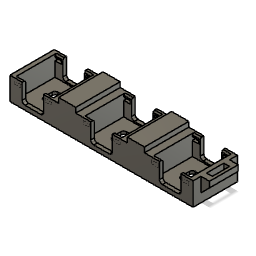
Magnet_Storage_Drawer (Autodesk Fusion 360 design; units mm, degrees)
Autodesk Fusion 360 part; units mm, degrees
sketch "base" plane through (0, 0, 0) normal (0, 1, 0) x (1, 0, 0)
  line L0 (-64, 15.5) -> (64, 15.5)
  line L1 (64, 15.5) -> (64, -15.5)
  line L2 (64, -15.5) -> (-64, -15.5)
  line L3 (-64, -15.5) -> (-64, 15.5)
  line L4 (64, 0) -> (-64, 0) construction
  line L5 (0, 15.5) -> (0, -15.5) construction
  line L6 (-61, 13) -> (-35, 13)
  line L7 (-35, 13) -> (-35, -13)
  line L8 (-35, -13) -> (-61, -13)
  line L9 (-61, -13) -> (-61, 13)
  line L10 (-53, 5) -> (-43, 5)
  line L11 (-43, 5) -> (-43, -5)
  line L12 (-43, -5) -> (-53, -5)
  line L13 (-53, -5) -> (-53, 5)
  line L14 (-48, 13) -> (-48, -13) construction
  line L15 (-13, 13) -> (13, 13)
  line L16 (-13, -13) -> (-13, 13)
  line L17 (13, -13) -> (-13, -13)
  line L18 (5, -5) -> (-5, -5)
  line L19 (-5, -5) -> (-5, 5)
  line L20 (-5, 5) -> (5, 5)
  line L21 (5, 5) -> (5, -5)
  line L22 (13, 13) -> (13, -13)
  line L23 (35, 13) -> (61, 13)
  line L24 (35, -13) -> (35, 13)
  line L25 (61, -13) -> (35, -13)
  line L26 (53, -5) -> (43, -5)
  line L27 (43, -5) -> (43, 5)
  line L28 (43, 5) -> (53, 5)
  line L29 (53, 5) -> (53, -5)
  line L30 (61, 13) -> (61, -13)
  dimension "d2" = 31
  dimension "d3" = 26
  dimension "d4" = 10
  dimension "d5" = 3
  dimension "d8" = 48
  dimension "d9" = 0
  dimension "d86" = 3
  constraint horizontal L0
  constraint vertical L1
  constraint horizontal L2
  constraint vertical L3
  constraint midpoint L1 L4.start
  constraint midpoint L3 L4.end
  constraint midpoint L0 L5.start
  constraint midpoint L2 L5.end
  constraint coincident origin L5
  constraint coincident origin L4
  constraint horizontal L6
  constraint vertical L7
  constraint horizontal L8
  constraint vertical L9
  constraint horizontal L10
  constraint vertical L11
  constraint horizontal L12
  constraint vertical L13
  constraint equal L6 L7
  constraint equal L10 L11
  constraint symmetric L4 L6 L8
  constraint midpoint L6 L14.start
  constraint midpoint L8 L14.end
  constraint symmetric L4 L10 L12
  constraint symmetric L11 L13 L14
  measures "d2" distance of L0.start L2.end
  measures "d3" distance of L6.start L8.end
  measures "d4" distance of L10.start L10.end
  measures "d5" distance of L3 L9
  measures "d86" distance of L1 L30
extrude "Extrude1" add sketch "base" along normal blind 2 contours L6 L7 L8 L9 | L15 L16 L17 L22 | L23 L24 L25 L30 makes body 1 at (10.3333, 0, -1.6667) makes body 2 at (58.3333, 0, 1.6667) makes body 3 at (-58.3333, 0, 1.6667)
extrude "Extrude2" add sketch "base" along normal blind 12 contours L0 L1 L2 L3 bodies 1 2 3
sketch "access slots" plane through (0, 0, 15.5) normal (0, 0, 1) x (1, 0, 0)
  line L0 (-64, 0) -> (64, 0)
  line L1 (64, 0) -> (64, 12)
  line L2 (64, 12) -> (-64, 12)
  line L3 (-64, 12) -> (-64, 0)
  line L4 (-42.5, 3) -> (-53.5, 3)
  line L5 (-55.5, 5) -> (-55.5, 12)
  line L6 (-55.5, 12) -> (-40.5, 12)
  line L7 (-40.5, 12) -> (-40.5, 5)
  line L8 (64, 0) -> (-64, 0)
  line L9 (-48, 12) -> (-48, 3) construction
  arc A0 (-55.5, 5) -> (-53.5, 3) centre (-53.5, 5) ccw
  arc A1 (-42.5, 3) -> (-40.5, 5) centre (-42.5, 5) ccw
  line L10 (-7.5, 5) -> (-7.5, 12)
  line L11 (-7.5, 12) -> (7.5, 12)
  arc A2 (-7.5, 5) -> (-5.5, 3) centre (-5.5, 5) ccw
  line L12 (5.5, 3) -> (-5.5, 3)
  arc A3 (5.5, 3) -> (7.5, 5) centre (5.5, 5) ccw
  line L13 (7.5, 12) -> (7.5, 5)
  line L14 (40.5, 5) -> (40.5, 12)
  line L15 (40.5, 12) -> (55.5, 12)
  arc A4 (40.5, 5) -> (42.5, 3) centre (42.5, 5) ccw
  line L16 (53.5, 3) -> (42.5, 3)
  arc A5 (53.5, 3) -> (55.5, 5) centre (53.5, 5) ccw
  line L17 (55.5, 12) -> (55.5, 5)
  point P0 (-61, 12)
  point P1 (-13, 12)
  point P2 (35, 12)
  point P3 (35, 15)
  dimension "d20" = 3
  dimension "d21" = 15
  dimension "d22" = 13
  dimension "d23" = 2
  dimension "d26" = 48
  dimension "d27" = 0
  constraint horizontal L4
  constraint vertical L5
  constraint horizontal L6
  constraint vertical L7
  constraint midpoint L6 L9.start
  constraint collinear L2 L6
  constraint coincident L4 L9.end
  constraint tangent L4 A0
  constraint tangent L5 A0
  constraint tangent L4 A1
  constraint tangent L7 A1
  constraint equal A0 A1
  constraint midpoint L4 L9.end
  measures "d20" distance of L4 L8
  measures "d21" distance of L5.end L6.end
  measures "d22" distance of P0 L9
  measures "d23" radius of A0
extrude "Extrude3" cut sketch "access slots" against normal up to surface (31 mm away) contours L2 L4 L5 L6 L7 A0 A1 | L2 L14 L15 A4 L16 A5 L17 | L2 L10 L11 A2 L12 A3 L13 bodies 1
fillet "Fillet1" radius 2 12 edges at (-43, 1, 5) (-53, 1, 5) (-53, 1, -5) (-43, 1, -5) (5, 1, -5) (5, 1, 5) (-5, 1, 5) (-5, 1, -5) (43, 1, -5) (43, 1, 5) (53, 1, -5) (53, 1, 5) on bodies 1
ref_plane "WorkPlane1" through (0, 12, 0) normal (0, 1, 0) x (0, 0, 1)
sketch "cover indents" plane through (-24, 12, 0) normal (0, 1, 0) x (1, 0, 0)
  circle A0 centre (-5, 9.5) radius 1.4
  circle A1 centre (-5, 9.5) radius 3
  line L0 (16.5, 15.5) -> (-16.5, 15.5)
  line L1 (-5, 12.5) -> (-11, 12.5)
  line L2 (11, -13) -> (-11, -13)
  circle A2 centre (5, 9.5) radius 1.4
  circle A3 centre (5, 9.5) radius 3
  line L3 (-5, 9.5) -> (5, 9.5) construction
  line L4 (5, 12.5) -> (11, 12.5)
  line L5 (-11, 13) -> (-11, -13)
  line L6 (11, -13) -> (11, 13)
  line L7 (-11, -13) -> (-16.5, -13)
  line L8 (-2, 9.5) -> (-2, 8)
  line L9 (2, 9.5) -> (2, 8)
  circle A4 centre (43, -9.5) radius 1.4
  circle A5 centre (43, -9.5) radius 3
  line L10 (37, 13) -> (37, -13)
  line L11 (31.5, -15.5) -> (64.5, -15.5)
  circle A6 centre (53, -9.5) radius 1.4
  circle A7 centre (53, -9.5) radius 3
  line L12 (43, -9.5) -> (53, -9.5) construction
  line L13 (59, -13) -> (59, 13) construction
  line L14 (43, -12.5) -> (37, -12.5)
  line L15 (59, -12.5) -> (53, -12.5)
  line L16 (37, 13) -> (59, 13)
  line L17 (37, 13) -> (37, -12.5)
  line L18 (59, -13) -> (59, 13)
  line L19 (46, -9.5) -> (46, -6.5)
  line L20 (46, -6.5) -> (50, -6.5)
  line L21 (50, -6.5) -> (50, -9.5)
  line L22 (-2, 8) -> (2, 8)
  dimension "d33" = 2.8
  dimension "d34" = 6
  dimension "d35" = 6
  dimension "d37" = 6
  dimension "d38" = 6
  dimension "d57" = 6
  dimension "d58" = 6
  dimension "d59" = 6
  dimension "d84" = 1.5
  constraint concentric A0 A1
  constraint coincident A1 L1.start
  constraint horizontal L1
  constraint equal A0 A2
  constraint concentric A2 A3
  constraint equal A1 A3
  constraint coincident A0.centre A1.centre
  constraint coincident A2.centre A3.centre
  constraint horizontal L3
  constraint coincident A3 L4.start
  constraint horizontal L4
  constraint coincident L4.end L6
  constraint coincident L1.end L5
  constraint tangent A1 L1
  constraint tangent A3 L4
  constraint coincident L2.end L5
  constraint coincident L2.start L6
  constraint collinear L2 L7
  constraint coincident A1 L8.start
  constraint coincident L3 L8.start
  constraint tangent A1 L8
  constraint coincident A3 L9.start
  constraint coincident L3 L9.start
  constraint tangent A3 L9
  constraint equal A2 A4
  constraint concentric A4 A5
  constraint equal A3 A5
  constraint concentric A6 A7
  constraint equal A4 A6
  constraint equal A5 A7
  constraint coincident A4.centre A5.centre
  constraint coincident A6.centre A7.centre
  constraint horizontal L12
  constraint coincident A5 L14.start
  constraint coincident L10 L14.end
  constraint tangent A5 L14
  constraint horizontal L14
  constraint coincident L13 L15.start
  constraint coincident A7 L15.end
  constraint perpendicular L13 L15
  constraint tangent A7 L15
  constraint coincident L10.start L16.start
  constraint coincident L13.end L16.end
  constraint coincident L13.start L18.start
  constraint coincident A5 L19.start
  constraint coincident L12 L19.start
  constraint tangent A5 L19
  constraint perpendicular L18 L20
  constraint coincident A7 L21.end
  constraint coincident L12 L21.end
  constraint tangent A7 L21
  constraint tangent A5 L20
  constraint equal L8 L9
  measures "d33" diameter of A0
  measures "d34" diameter of A1
  measures "d35" distance of A0.centre L0
  measures "d37" distance of A0.centre L5
  measures "d38" distance of A2.centre L6
  measures "d57" distance of A4.centre L10
  measures "d58" distance of A4.centre L11
  measures "d59" distance of A6.centre L13
  measures "d84" distance of L9.start L9.end
extrude "Extrude9" add 2 faces at (-63, 12, -4.3333) (63, 12, 4.3333) along direction (0, 1, 0) blind 4 on bodies 1 bodies 1
sketch "left top" plane through (0, 12, 0) normal (0, 1, 0) x (-1, 0, 0)
  line L0 (-7.5, -15.5) -> (-7.5, -13)
  line L1 (-7.5, -13) -> (-13, -13)
  line L2 (-13, -13) -> (-13, 13)
  line L3 (-13, 13) -> (-7.5, 13)
  line L4 (-7.5, 13) -> (-7.5, 15.5)
  line L5 (-7.5, 15.5) -> (-40.5, 15.5)
  line L6 (-40.5, 15.5) -> (-40.5, 13)
  line L7 (-40.5, 13) -> (-35, 13)
  line L8 (-35, 13) -> (-35, -13)
  line L9 (-35, -13) -> (-40.5, -13)
  line L10 (-40.5, -13) -> (-40.5, -15.5)
  line L11 (-40.5, -15.5) -> (-7.5, -15.5)
  line L12 (-30, 15.5) -> (-30, -15.5)
  line L13 (-18, 15.5) -> (-18, -15.5)
  dimension "d94" = 5
  dimension "d95" = 5
  dimension "d138" = 12
  constraint coincident L5 L12.start
  constraint coincident L11 L12.end
  constraint perpendicular L11 L12
  constraint coincident L5 L13.start
  constraint coincident L11 L13.end
  constraint perpendicular L11 L13
  measures "d94" distance of L8 L12
  measures "d95" distance of L2 L13
  measures "d138" distance of L12 L13
extrude "Extrude11" add sketch "left top" along normal blind 4 contours L5 L6 L7 L8 L9 L10 L11 L12 bodies 1
ref_plane "WorkPlane4" through (48, 9, 13) normal (0, 0, -1) x (-1, 0, 0)
sketch "left prong holes" plane through (37.75, 13.75, 13) normal (0, 0, -1) x (1, 0, 0)
  line L0 (1.75, -0.25) -> (-2.75, -0.25)
  line L1 (-2.75, -0.25) -> (-2.75, 2)
  line L2 (-2.75, 2) -> (1.75, 2)
  line L3 (1.75, 2) -> (1.75, -0.25)
  line L4 (2.75, -2.25) -> (2.75, 8.75)
  line L5 (18.75, -0.25) -> (23.25, -0.25)
  line L6 (23.25, -0.25) -> (23.25, 2)
  line L7 (23.25, 2) -> (18.75, 2)
  line L8 (18.75, 2) -> (18.75, -0.25)
  line L9 (17.75, 8.75) -> (17.75, -2.25)
  line L10 (-7.75, -2.25) -> (2.75, -2.25)
  line L11 (17.75, -2.25) -> (26.25, -2.25)
  dimension "d119" = 1
  dimension "d120" = 4.5
  dimension "d121" = 2.25
  dimension "d123" = 1
  dimension "d125" = 2.25
  dimension "d132" = 2
  dimension "d133" = 2
  constraint horizontal L0
  constraint vertical L1
  constraint horizontal L2
  constraint vertical L3
  constraint horizontal L5
  constraint vertical L6
  constraint horizontal L7
  constraint vertical L8
  constraint equal L0 L5
  measures "d119" distance of L3 L4
  measures "d120" distance of L0.start L0.end
  measures "d121" distance of L0.end L1.end
  measures "d123" distance of L8 L9
  measures "d125" distance of L5.start L7.end
  measures "d132" distance of L0 L10
  measures "d133" distance of L5 L11
extrude "Extrude16" cut sketch "left prong holes" against normal blind 2 bodies 1
mirror "Mirror1" about plane through (0, 0, 0) normal (0, 0, 1) of "Extrude16"
sketch "right top" plane through (0, 12, 0) normal (0, 1, 0) x (-1, 0, 0)
  line L0 (40.5, -15.5) -> (40.5, -13)
  line L1 (40.5, -13) -> (35, -13)
  line L2 (35, -13) -> (35, 13)
  line L3 (35, 13) -> (40.5, 13)
  line L4 (40.5, 13) -> (40.5, 15.5)
  line L5 (40.5, 15.5) -> (7.5, 15.5)
  line L6 (7.5, 15.5) -> (7.5, 13)
  line L7 (7.5, 13) -> (13, 13)
  line L8 (13, 13) -> (13, -13)
  line L9 (13, -13) -> (7.5, -13)
  line L10 (7.5, -13) -> (7.5, -15.5)
  line L11 (7.5, -15.5) -> (40.5, -15.5)
  line L12 (18, 15.5) -> (18, -15.5)
  line L13 (30, 15.5) -> (30, -15.5)
  dimension "d141" = 5
  dimension "d142" = 5
  constraint coincident L5 L12.start
  constraint coincident L11 L12.end
  constraint perpendicular L11 L12
  constraint coincident L5 L13.start
  constraint coincident L11 L13.end
  constraint perpendicular L11 L13
  measures "d141" distance of L8 L12
  measures "d142" distance of L2 L13
extrude "Extrude17" add sketch "right top" sketch "left top" along normal blind 7.5 contours L5 L11 L12 L13 of sketch 2 contours L5 L11 L12 L13 bodies 1
extrude "Extrude18" add sketch "left top" 2 faces at (-16.3333, 12, -4.3333) (-31.6667, 12, 4.3333) along normal blind 4 contours L0 L1 L2 L3 L4 L5 L11 L13 on bodies 1 bodies 1
sketch "middle prong holes" plane through (0, 0, 13) normal (0, 0, -1) x (-1, 0, 0)
  line L0 (-7.5, 5) -> (-7.5, 16)
  line L1 (-7.5, 16) -> (-13, 16)
  line L2 (-13, 16) -> (-13, 2)
  line L3 (-13, 2) -> (13, 2)
  line L4 (13, 2) -> (13, 16)
  line L5 (13, 16) -> (7.5, 16)
  line L6 (7.5, 16) -> (7.5, 5)
  arc A0 (5.5, 3) -> (7.5, 5) centre (5.5, 5) ccw
  line L7 (5.5, 3) -> (-5.5, 3)
  arc A1 (-7.5, 5) -> (-5.5, 3) centre (-5.5, 5) ccw
  line L8 (-13, 14) -> (-8.5, 14)
  line L9 (-8.5, 14) -> (-8.5, 12)
  line L10 (-8.5, 12) -> (-13, 12)
  line L11 (-13, 12) -> (-13, 14)
  line L12 (8.5, 14) -> (13, 14)
  line L13 (13, 14) -> (13, 12)
  line L14 (13, 12) -> (8.5, 12)
  line L15 (8.5, 12) -> (8.5, 14)
  dimension "d145" = 2
  dimension "d146" = 1
  dimension "d147" = 4.5
  dimension "d148" = 2
  dimension "d149" = 1
  constraint horizontal L8
  constraint vertical L9
  constraint horizontal L10
  constraint vertical L11
  constraint horizontal L12
  constraint vertical L13
  constraint horizontal L14
  constraint vertical L15
  constraint collinear L8 L12
  constraint collinear L10 L14
  constraint equal L8 L12
  measures "d145" distance of L1 L8
  measures "d146" distance of L0 L9
  measures "d147" distance of L8.start L8.end
  measures "d148" distance of L8.end L9.end
  measures "d149" distance of L6 L15
sketch "right prong holes" plane through (0, 0, 13) normal (0, 0, -1) x (-1, 0, 0)
  line L0 (40.5, 5) -> (40.5, 16)
  line L1 (40.5, 16) -> (35, 16)
  line L2 (35, 16) -> (35, 2)
  line L3 (35, 2) -> (61, 2)
  line L4 (61, 2) -> (61, 16)
  line L5 (61, 16) -> (55.5, 16)
  line L6 (55.5, 16) -> (55.5, 5)
  arc A0 (53.5, 3) -> (55.5, 5) centre (53.5, 5) ccw
  line L7 (53.5, 3) -> (42.5, 3)
  arc A1 (40.5, 5) -> (42.5, 3) centre (42.5, 5) ccw
  line L8 (35, 14) -> (39.5, 14)
  line L9 (39.5, 14) -> (39.5, 12)
  line L10 (39.5, 12) -> (35, 12)
  line L11 (35, 12) -> (35, 14)
  line L12 (56.5, 14) -> (61, 14)
  line L13 (61, 14) -> (61, 12)
  line L14 (61, 12) -> (56.5, 12)
  line L15 (56.5, 12) -> (56.5, 14)
  dimension "d150" = 1
  dimension "d151" = 2
  dimension "d152" = 4.5
  dimension "d153" = 2
  dimension "d154" = 1
  constraint horizontal L8
  constraint vertical L9
  constraint horizontal L10
  constraint vertical L11
  constraint horizontal L12
  constraint vertical L13
  constraint horizontal L14
  constraint vertical L15
  constraint equal L8 L12
  constraint collinear L8 L12
  constraint collinear L10 L14
  measures "d150" distance of L0 L9
  measures "d151" distance of L1 L8
  measures "d152" distance of L8.start L8.end
  measures "d153" distance of L8.end L9.end
  measures "d154" distance of L6 L15
extrude "Extrude19" cut sketch "middle prong holes" sketch "right prong holes" along normal blind 28 and the other way blind 2 contours L2 L8 L9 L10 L11 | L4 L12 L13 L14 L15 of sketch 2 contours L2 L8 L9 L10 L11 | L4 L12 L13 L14 L15 bodies 1
chamfer "Chamfer2" distance 1 angle 45 2 edges at (37.75, 16, 13) (58.25, 16, 13) on bodies 1
chamfer "Chamfer2" distance 1 angle 45 2 edges at (37.75, 16, -13) (58.25, 16, -13) on bodies 1
chamfer "Chamfer2" distance 1 angle 45 8 edges at (10.25, 16, 13) (-10.25, 16, 13) (10.25, 16, -13) (-10.25, 16, -13) (-37.75, 16, 13) (-58.25, 16, 13) (-58.25, 16, -13) (-37.75, 16, -13) on bodies 1
sketch "handle" plane through (64, 0, 0) normal (1, 0, 0) x (0, 0, -1)
  line L0 (-15.5, 0) -> (15.5, 0)
  line L1 (15.5, 0) -> (15.5, 16)
  line L2 (-15.5, 16) -> (-15.5, 0)
  line L3 (-10, 16) -> (10, 16)
  line L4 (10, 16) -> (10, 12)
  line L5 (10, 12) -> (-10, 12)
  line L6 (-10, 12) -> (-10, 16)
  line L7 (0, 19) -> (0, 0) construction
  line L8 (-6, 16) -> (-6, 12)
  line L9 (6, 16) -> (6, 12)
  line L10 (15.5, 16) -> (-15.5, 16)
  dimension "d73" = 20
  dimension "d74" = 4
  dimension "d76" = 4
  dimension "d77" = 4
  constraint horizontal L3
  constraint vertical L4
  constraint horizontal L5
  constraint vertical L6
  constraint coincident L7.end origin
  constraint symmetric L4 L6 L7
  constraint coincident L3 L8.start
  constraint coincident L5 L8.end
  constraint perpendicular L5 L8
  constraint coincident L3 L9.start
  constraint coincident L5 L9.end
  constraint perpendicular L5 L9
  measures "d73" distance of L3.start L3.end
  measures "d74" distance of L3.start L5.end
  measures "d76" distance of L4 L9
  measures "d77" distance of L6 L8
extrude "Extrude7" add sketch "handle" along normal blind 6 contours L3 L5 L6 L8 L10 | L3 L4 L5 L9 L10 | L3 L5 L8 L9 L10 bodies 1
extrude "Extrude8" cut sketch "handle" along normal blind 4 contours L3 L5 L8 L9 L10 bodies 1
draft "Draft1" angle 45 neutral plane through (70, 0, 0) pull (1, 0, 0) 1 faces at (67.3333, 12, -8.6667) on bodies 1
equation "d38 = d37"
equation "d57 = d37"
equation "d58 = d35"
equation "d59 = d37"
equation "d77 = d76"
equation "d95 = d94"
equation "d123 = d119"
equation "d142 = d141"
equation "d149 = d146"
equation "d154 = d150"
